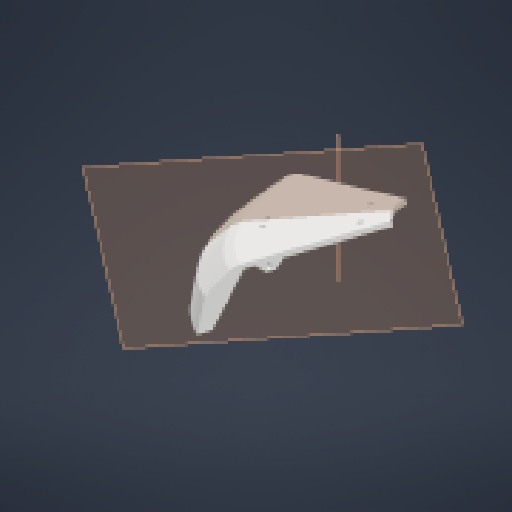
# Autodesk Inventor part: Head_BottomRight
Saved by Autodesk Inventor 2024 (Build 280153000, 153)
## iProperties
Created: 2025-09-16
Part Number: Head_BottomRight
Material: Generic
Document SubType Name: Modeling
Designer: kevin
Density: 1 g/cm^3
Appearance: Default
Author: kevin
Autodesk Inventor part; units mm, degrees
ref_plane "YZ Plane" through (0, 0, 0) normal (1, 0, 0) x (0, 1, 0)
ref_plane "XZ Plane" through (0, 0, 0) normal (0, 1, 0) x (-1, 0, 0)
ref_plane "XY Plane" through (0, 0, 0) normal (0, 0, 1) x (1, 0, 0)
sketch "Sketch1" plane through (0, 0, 0) normal (0, 0, 1) x (1, 0, 0)
  circle A0 centre (53.3917, 8.373) radius 2.1 projected
  line L0 (129.8213, 34.1894) -> (128.4206, 38.9296) projected
  line L1 (127.5739, 38.7084) -> (128.4206, 38.9296) projected
  line L2 (127.8489, 37.7776) -> (127.5739, 38.7084) projected
  line L3 (34.1095, 10.0789) -> (127.8489, 37.7776) projected
  line L4 (27.6493, 5.9265) -> (34.1095, 10.0789) projected
  line L5 (27.6493, 5.9265) -> (13.0395, -10.8812) projected
  line L6 (10.6122, -35.9144) -> (13.0395, -10.8812) projected
  line L7 (20.2023, -33.0807) -> (10.6122, -35.9144) projected
  line L8 (36.8802, 6.7266) -> (20.2023, -33.0807) projected
  line L9 (44.0002, 8.8305) -> (36.8802, 6.7266) projected
  line L10 (51.2014, 4.4933) -> (44.0002, 8.8305) projected
  line L11 (57.339, 6.3069) -> (51.2014, 4.4933) projected
  line L12 (61.3422, 13.9548) -> (57.339, 6.3069) projected
  line L13 (129.8213, 34.1894) -> (61.3422, 13.9548) projected
  line L14 (158.2559, 42.5914) -> (18.4899, 1.2925) projected
  line L15 (34.1095, 10.0789) -> (128.6878, 38.0254)
  line L16 (160.2698, 43.1865) -> (155.9107, 57.9387)
  point P0 (0, 0)
  constraints: 4 end point, 1 parallel, 1 perpendicular, 1 point on line
revolve "Revolution1" add sketch "Sketch1" angle 60 about axis through (160.2698, 43.1865, 0) along (-0.2834, 0.959, 0) contours L13 L14 L9 L5 L4 L3 L15 L0 | L8 L7 L6 L5 L14
ref_plane "Work Plane1" through (0, 0, 0) normal (0, 0, 1) x (1, 0, 0)
sketch "Sketch2" plane through (0, 0, 0) normal (0, 0, 1) x (1, 0, 0)
  circle A0 centre (53.3917, 8.373) radius 2.1 projected
  line L0 (129.8213, 34.1894) -> (128.4206, 38.9296) projected
  line L1 (127.5739, 38.7084) -> (128.4206, 38.9296) projected
  line L2 (127.8489, 37.7776) -> (127.5739, 38.7084) projected
  line L3 (34.1095, 10.0789) -> (127.8489, 37.7776) projected
  line L4 (27.6493, 5.9265) -> (34.1095, 10.0789) projected
  line L5 (27.6493, 5.9265) -> (13.0395, -10.8812) projected
  line L6 (10.6122, -35.9144) -> (13.0395, -10.8812) projected
  line L7 (20.2023, -33.0807) -> (10.6122, -35.9144) projected
  line L8 (36.8802, 6.7266) -> (20.2023, -33.0807) projected
  line L9 (44.0002, 8.8305) -> (36.8802, 6.7266) projected
  line L10 (51.2014, 4.4933) -> (44.0002, 8.8305) projected
  line L11 (57.339, 6.3069) -> (51.2014, 4.4933) projected
  line L12 (61.3422, 13.9548) -> (57.339, 6.3069) projected
  line L13 (129.8213, 34.1894) -> (61.3422, 13.9548) projected
  line L14 (158.2559, 42.5914) -> (18.4899, 1.2925) projected
  point P0 (0, 0)
extrude "Extrusion1" add sketch "Sketch2" along normal blind 7 contours L12 L11 L10 L14
sketch "Sketch3" plane through (61.3422, 13.9548, 0) normal (0.2834, -0.959, 0) x (0.959, 0.2834, 0)
  circle A0 centre (4.1416, 56.7109) radius 2.1
  circle A1 centre (9.1416, 65.8342) radius 2.1
  circle A2 centre (68.5106, 37.1528) radius 2.1 projected
  circle A3 centre (54.5758, 14.8525) radius 2.1 projected
  point P0 (-62.7821, 0)
  dimension "d3" = 4.2
  dimension "d4" = 4.2
  dimension "d5" = 5
  constraints: 2 centre point
  measures "d3" diameter of A0
  measures "d4" diameter of A1
  measures "d5" horizontal distance of A1.centre A0.centre
extrude "Extrusion2" cut sketch "Sketch3" against normal blind 7
ref_plane "Work Plane2" through (159.1363, 47.0226, 0) normal (0.4795, 0.1417, 0.866) x (0.2834, -0.959, 0)
mirror "Mirror1" about plane through (159.1363, 47.0226, 0) normal (0.4795, 0.1417, 0.866) of "Extrusion1"
body "Solid1"
